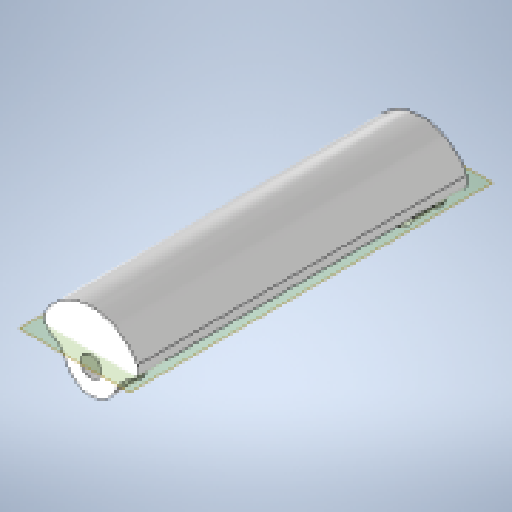
# Autodesk Inventor part: Front Bumper
Saved by Autodesk Inventor 2023.2 (Build 272271000, 271)
## iProperties
Created: 2024-04-05
Part Number: Front Bumper
Material: Nylon 6/6
Document SubType Name: Modeling
Designer: Nathan Cai
Density: 1.13 g/cm^3
Appearance: Smooth - White
Mass: 4.07406 g
Surface Area: 21.8418 cm^2
Volume: 3.60536 cm^3
Author: Nathan Cai
Autodesk Inventor part; units mm, degrees
ref_plane "YZ Plane" through (0, 0, 0) normal (1, 0, 0) x (0, 1, 0)
ref_plane "XZ Plane" through (0, 0, 0) normal (0, 1, 0) x (-1, 0, 0)
ref_plane "XY Plane" through (0, 0, 0) normal (0, 0, 1) x (1, 0, 0)
sketch "Sketch1" plane through (0, 0, 0) normal (0, 0, 1) x (1, 0, 0)
  circle A0 centre (0, 0) radius 1.5875
  circle A1 centre (0, 0) radius 8
  line L0 (0, 0) -> (0, 8) construction
  line L1 (1.5334, 0.4109) -> (7.7274, 2.0706)
  line L2 (-1.5334, 0.4109) -> (-7.7274, 2.0706)
  circle A2 centre (0, 0) radius 3.9688
  point P0 (-3.8335, 1.0272)
  point P1 (3.8335, 1.0272)
  dimension "d0" = 3.175
  dimension "d1" = 16
  dimension "d2" = 75
  dimension "d3" = 7.9375
  constraints: 6 end point, 3 coincident, 2 centre point, 2 point on circle, 2 symmetric about line, 1 point on line, 1 vertical, 3 other
  measures "d1" diameter of A1
  measures "d2" angle of L0 L1
  measures "d3" diameter of A2
extrude "Extrusion1" add sketch "Sketch1" along normal blind 50.8 contours A0 L1 A2 L2 | A0 L2 A2 L1 | A2 L2 A1 L1 picked at (6.1941, 2.3106)
fillet "Fillet1" radius 3.175 2 edges at (-3.8335, 1.0272, 25.4) (3.8335, 1.0272, 25.4)
ref_plane "Work Plane1" through (7.7274, 2.0706, 0) normal (0, -1, 0) x (0, 0, 1)
sketch "Sketch2" plane through (7.7274, 2.0706, 0) normal (0, -1, 0) x (0, 0, 1)
  line L0 (0, 15.4548) -> (50.8, 15.4548) projected
  line L1 (25.4, 15.4548) -> (25.4, 0) construction
  line L2 (0, 0) -> (50.8, 0) projected
  line L3 (0, 7.7274) -> (50.8, 7.7274) construction
  line L4 (50.8, 9.3149) -> (50.8, 6.1399) projected
  line L5 (36.5125, 0) -> (46.0375, 0)
  line L6 (46.0375, 0) -> (46.0375, 15.4548)
  line L7 (46.0375, 15.4548) -> (36.5125, 15.4548)
  line L8 (36.5125, 15.4548) -> (36.5125, 0)
  line L9 (36.5125, 0) -> (46.0375, 15.4548) construction
  line L10 (46.0375, 0) -> (36.5125, 15.4548) construction
  line L11 (50.8, 11.618) -> (50.8, 15.4548) projected
  line L12 (14.2875, 0) -> (4.7625, 0)
  line L13 (4.7625, 0) -> (4.7625, 15.4548)
  line L14 (4.7625, 15.4548) -> (14.2875, 15.4548)
  line L15 (14.2875, 15.4548) -> (14.2875, 0)
  line L16 (14.2875, 0) -> (4.7625, 15.4548) construction
  line L17 (4.7625, 0) -> (14.2875, 15.4548) construction
  point P0 (41.275, 7.7274)
  point P1 (9.525, 7.7274)
  point P2 (46.0375, 0)
  point P3 (4.7625, 0)
  dimension "d7" = 4.7625
  dimension "d8" = 9.525
  constraints: 28 end point, 5 midpoint, 5 symmetric about line, 2 parallel, 2 point on line, 1 horizontal, 1 perpendicular
  measures "d7" distance between parallel lines of L11 L6
  measures "d8" distance between parallel lines of L8 L6
extrude "Extrusion2" cut sketch "Sketch2" along normal blind 12.0904 and the other way blind 0.254
fillet "Fillet2" radius 1.5875 3 edges at (-7.7274, 2.0706, 2.3813) (-7.7274, 2.0706, 48.4187) (7.7274, 2.0706, 2.3813)
body "Solid1"
